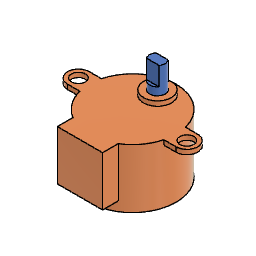
Zen_Garden_Model (Autodesk Fusion 360 archive; units mm, degrees)
design "Stepper motor"
Autodesk Fusion 360 part; units mm, degrees
sketch "Sketch1" plane through (0, 0, 0) normal (0, 0, 1) x (1, 0, 0)
  circle A0 centre (0, 0) radius 14
  dimension "d151" = 28
  constraint coincident A0.centre origin
  measures "d151" diameter of A0
extrude "Extrude1" add sketch "Sketch1" along normal blind 19 makes body 1
sketch "Sketch6" plane through (0, 0, 19) normal (0, 0, 1) x (-1, 0, 0)
  circle A0 centre (0, 0) radius 14
  circle A1 centre (0, -8) radius 4.5
  line L0 (-21, -3.5) -> (21, -3.5)
  line L1 (21, -3.5) -> (21, 3.5)
  line L2 (21, 3.5) -> (-21, 3.5)
  line L3 (-21, 3.5) -> (-21, -3.5)
  line L4 (-21, -3.5) -> (21, 3.5) construction
  line L5 (21, -3.5) -> (-21, 3.5) construction
  circle A2 centre (17.5, 0) radius 3.5
  circle A3 centre (17.5, 0) radius 2.25
  line L6 (0, 0) -> (0, -17) construction
  circle A4 centre (-17.5, 0) radius 3.5
  circle A5 centre (-17.5, 0) radius 2.25
  line L7 (7.3, 0) -> (-7.3, 0)
  line L8 (-7.3, 0) -> (-7.3, 17)
  line L9 (-7.3, 17) -> (7.3, 17)
  line L10 (7.3, 17) -> (7.3, 0)
  dimension "d563" = 9
  dimension "d564" = 8
  dimension "d565" = 7
  dimension "d566" = 4.5
  dimension "d567" = 35
  dimension "d581" = 17
  dimension "d582" = 14.6
  constraint vertical A0.centre A1.centre
  constraint horizontal L0
  constraint perpendicular L0 L1
  constraint parallel L0 L2
  constraint parallel L1 L3
  constraint coincident L4 A0.centre
  constraint coincident L5 A0.centre
  constraint coincident A0.centre L6.start
  constraint tangent L0 A2
  constraint tangent L1 A2
  constraint concentric A2 A3
  constraint perpendicular L0 L6
  constraint symmetric A2 L6 A4
  constraint symmetric A3 L6 A5
  constraint tangent L2 A2
  constraint horizontal L7
  constraint vertical L8
  constraint horizontal L9
  constraint vertical L10
  constraint midpoint A0.centre L7
  measures "d563" diameter of A1
  measures "d564" distance of A0.centre A1.centre
  measures "d565" diameter of A2
  measures "d566" diameter of A3
  measures "d567" distance of A2.centre A4.centre
  measures "d581" distance of L7.end L8.end
  measures "d582" distance of L7.start L7.end
extrude "Extrude6" add sketch "Sketch6" along normal blind 1.5 contours A1 bodies 1
sketch "Sketch7" plane through (0, 0, 20.5) normal (0, 0, 1) x (-1, 0, 0)
  circle A0 centre (0, -8) radius 4.5
  circle A1 centre (0, -8) radius 2.5
  line L0 (2.5, -9.5) -> (-2.5, -9.5)
  line L1 (-2.5, -9.5) -> (-2.5, -6.5)
  line L2 (-2.5, -6.5) -> (2.5, -6.5)
  line L3 (2.5, -6.5) -> (2.5, -9.5)
  line L4 (2.5, -9.5) -> (-2.5, -6.5) construction
  line L5 (2.5, -6.5) -> (-2.5, -9.5) construction
  circle A2 centre (0, -8) radius 3.5
  dimension "d570" = 5
  dimension "d571" = 3
  dimension "d679" = 1
  constraint concentric A0 A1
  constraint horizontal L0
  constraint vertical L1
  constraint horizontal L2
  constraint vertical L3
  constraint tangent A1 L3
  constraint tangent A1 L1
  constraint coincident A0.centre L5
  constraint concentric A1 A2
  measures "d570" diameter of A1
  measures "d571" distance of L0.end L1.end
  measures "d679" distance of A1 A2
extrude "Extrude9" add sketch "Sketch6" against normal blind 1.5 contours A0 L0 A2 | A0 L2 A2 | A2 | A0 L0 A4 | A0 L2 A4 | A4 bodies 1
extrude "Extrude10" add sketch "Sketch6" against normal blind 16 contours A0 L8 L9 L10 bodies 1
extrude "Extrude1'" add sketch "Sketch7" along normal blind 2.5 separate body contours A1 L0 L2 | A1 L2 | A1 L0 makes body 2 in component "Axis"
extrude "Extrude2" add sketch "Sketch7" along normal up to surface (8.5 mm away) contours A1 L0 L2 bodies 2 in component "Axis"
component "Axis" placed x (1, 0, 0) y (0, 1, 0) z (0, 0, 1) at (0, 0, 0)
equation "d151 = motor_diameter"
equation "d152 = motor_heigth"
equation "motor_diameter = 28 mm"
equation "motor_heigth = 19 mm"
